Autodesk Fusion 360 part; units mm, degrees
(part 3 of 6)
ref_plane "WorkPlane5" through (73.27, 0, 0) normal (1, 0, 0) x (0, 1, 0) in component "USB — removable metal faceplate — local 1.80 mm seat"
sketch "GCT 9.64 x 3.86 gasket seat R1.65 profile" plane through (73.27, 0, 0) normal (1, 0, 0) x (0, 0, -1) in component "USB — removable metal faceplate — local 1.80 mm seat"
  line L0 (-25.07, 12.83) -> (-25.07, 19.17)
  arc A0 (-25.07, 19.17) -> (-26.72, 20.82) centre (-26.72, 19.17) ccw
  line L1 (-26.72, 20.82) -> (-27.28, 20.82)
  arc A1 (-27.28, 20.82) -> (-28.93, 19.17) centre (-27.28, 19.17) ccw
  line L2 (-28.93, 19.17) -> (-28.93, 12.83)
  arc A2 (-28.93, 12.83) -> (-27.28, 11.18) centre (-27.28, 12.83) ccw
  line L3 (-27.28, 11.18) -> (-26.72, 11.18)
  arc A3 (-26.72, 11.18) -> (-25.07, 12.83) centre (-26.72, 12.83) ccw
extrude "GCT 9.64 x 3.86 gasket seat R1.65" cut sketch "GCT 9.64 x 3.86 gasket seat R1.65 profile" along normal blind 0.5 bodies 36 in component "USB — removable metal faceplate — local 1.80 mm seat"
ref_plane "WorkPlane6" through (73.77, 0, 0) normal (1, 0, 0) x (0, 1, 0) in component "USB — removable metal faceplate — local 1.80 mm seat"
sketch "GCT throat at 0.67 mm from inner panel" plane through (73.77, 0, 0) normal (1, 0, 0) x (0, 0, -1) in component "USB — removable metal faceplate — local 1.80 mm seat"
  line L0 (-25.67, 12.83) -> (-25.67, 19.17)
  arc A0 (-25.67, 19.17) -> (-26.72, 20.22) centre (-26.72, 19.17) ccw
  line L1 (-26.72, 20.22) -> (-27.28, 20.22)
  arc A1 (-27.28, 20.22) -> (-28.33, 19.17) centre (-27.28, 19.17) ccw
  line L2 (-28.33, 19.17) -> (-28.33, 12.83)
  arc A2 (-28.33, 12.83) -> (-27.28, 11.78) centre (-27.28, 12.83) ccw
  line L3 (-27.28, 11.78) -> (-26.72, 11.78)
  arc A3 (-26.72, 11.78) -> (-25.67, 12.83) centre (-26.72, 12.83) ccw
ref_plane "WorkPlane7" through (74.9, 0, 0) normal (1, 0, 0) x (0, 1, 0) in component "USB — removable metal faceplate — local 1.80 mm seat"
sketch "GCT nominal 10-degree external lead-in" plane through (74.9, 0, 0) normal (1, 0, 0) x (0, 0, -1) in component "USB — removable metal faceplate — local 1.80 mm seat"
  line L0 (-25.4708, 12.83) -> (-25.4708, 19.17)
  arc A0 (-25.4708, 19.17) -> (-26.72, 20.4192) centre (-26.72, 19.17) ccw
  line L1 (-26.72, 20.4192) -> (-27.28, 20.4192)
  arc A1 (-27.28, 20.4192) -> (-28.5292, 19.17) centre (-27.28, 19.17) ccw
  line L2 (-28.5292, 19.17) -> (-28.5292, 12.83)
  arc A2 (-28.5292, 12.83) -> (-27.28, 11.5808) centre (-27.28, 12.83) ccw
  line L3 (-27.28, 11.5808) -> (-26.72, 11.5808)
  arc A3 (-26.72, 11.5808) -> (-25.4708, 12.83) centre (-26.72, 12.83) ccw
loft "GCT reference tapered entry cutting tool" add profiles "GCT throat at 0.67 mm from inner panel", "GCT nominal 10-degree external lead-in" section 1 section 2 separate body makes body 38 in component "USB — removable metal faceplate — local 1.80 mm seat"
combine "Nominal 10-degree USB entry" operation cut target body 36 tool bodies 38 in component "USB — removable metal faceplate — local 1.80 mm seat"
ref_plane "WorkPlane3" through (0, 0, 22.7) normal (0, 0, 1) x (1, 0, 0) in component "USB — removable panel insert and board supports"
sketch "USB board support rail sketch" plane through (0, 0, 22.7) normal (0, 0, 1) x (1, 0, 0) in component "USB — removable panel insert and board supports"
  line L0 (60.1, 8) -> (70.6, 8)
  line L1 (70.6, 8) -> (70.6, 11.6)
  line L2 (70.6, 11.6) -> (60.1, 11.6)
  line L3 (60.1, 11.6) -> (60.1, 8)
  dimension "d962" = 60.1
  dimension "d963" = 8
  dimension "d964" = 10.5
  dimension "d965" = 3.6
  constraint horizontal L0
  constraint vertical L1
  constraint horizontal L2
  constraint vertical L3
  measures "d962" horizontal distance of origin L0.start
  measures "d963" vertical distance of origin L0.start
  measures "d964" horizontal distance of L0.start L0.end
  measures "d965" vertical distance of L0.end L1.end
extrude "USB board support rail" add sketch "USB board support rail sketch" along normal blind 4 bodies 37 in component "USB — removable panel insert and board supports"
ref_plane "WorkPlane4" through (0, 0, 22.7) normal (0, 0, 1) x (1, 0, 0) in component "USB — removable panel insert and board supports"
sketch "USB board M2 support boss sketch" plane through (0, 0, 22.7) normal (0, 0, 1) x (1, 0, 0) in component "USB — removable panel insert and board supports"
  circle A0 centre (63.7, 10.4) radius 3.6
  dimension "d970" = 63.7
  dimension "d971" = 10.4
  dimension "d972" = 3.6
  measures "d970" horizontal distance of origin A0.centre
  measures "d971" vertical distance of origin A0.centre
  measures "d972" radius of A0
extrude "USB board M2 support boss" add sketch "USB board M2 support boss sketch" along normal blind 4 bodies 37 in component "USB — removable panel insert and board supports"
ref_plane "WorkPlane5" through (0, 0, 22.6) normal (0, 0, 1) x (1, 0, 0) in component "USB — removable panel insert and board supports"
sketch "USB board insert pilot reference sketch" plane through (0, 0, 22.6) normal (0, 0, 1) x (1, 0, 0) in component "USB — removable panel insert and board supports"
  circle A0 centre (63.7, 10.4) radius 1.6
  dimension "d977" = 63.7
  dimension "d978" = 10.4
  dimension "d979" = 1.6
  measures "d977" horizontal distance of origin A0.centre
  measures "d978" vertical distance of origin A0.centre
  measures "d979" radius of A0
extrude "USB board insert pilot reference" cut sketch "USB board insert pilot reference sketch" along normal blind 4.2 bodies 37 in component "USB — removable panel insert and board supports"
ref_plane "WorkPlane6" through (0, 0, 22.7) normal (0, 0, 1) x (1, 0, 0) in component "USB — removable panel insert and board supports"
sketch "USB board support rail sketch (1)" plane through (0, 0, 22.7) normal (0, 0, 1) x (1, 0, 0) in component "USB — removable panel insert and board supports"
  line L0 (57.5, 20.4) -> (70.6, 20.4)
  line L1 (70.6, 20.4) -> (70.6, 24)
  line L2 (70.6, 24) -> (57.5, 24)
  line L3 (57.5, 24) -> (57.5, 20.4)
  dimension "d984" = 57.5
  dimension "d985" = 20.4
  dimension "d986" = 13.1
  dimension "d987" = 3.6
  constraint horizontal L0
  constraint vertical L1
  constraint horizontal L2
  constraint vertical L3
  measures "d984" horizontal distance of origin L0.start
  measures "d985" vertical distance of origin L0.start
  measures "d986" horizontal distance of L0.start L0.end
  measures "d987" vertical distance of L0.end L1.end
extrude "USB board support rail (1)" add sketch "USB board support rail sketch (1)" along normal blind 4 bodies 37 in component "USB — removable panel insert and board supports"
ref_plane "WorkPlane7" through (0, 0, 22.7) normal (0, 0, 1) x (1, 0, 0) in component "USB — removable panel insert and board supports"
sketch "USB board M2 support boss sketch (1)" plane through (0, 0, 22.7) normal (0, 0, 1) x (1, 0, 0) in component "USB — removable panel insert and board supports"
  circle A0 centre (59.5, 21.6) radius 3.6
  dimension "d992" = 59.5
  dimension "d993" = 21.6
  dimension "d994" = 3.6
  measures "d992" horizontal distance of origin A0.centre
  measures "d993" vertical distance of origin A0.centre
  measures "d994" radius of A0
extrude "USB board M2 support boss (1)" add sketch "USB board M2 support boss sketch (1)" along normal blind 4 bodies 37 in component "USB — removable panel insert and board supports"
ref_plane "WorkPlane8" through (0, 0, 22.6) normal (0, 0, 1) x (1, 0, 0) in component "USB — removable panel insert and board supports"
sketch "USB board insert pilot reference sketch (1)" plane through (0, 0, 22.6) normal (0, 0, 1) x (1, 0, 0) in component "USB — removable panel insert and board supports"
  circle A0 centre (59.5, 21.6) radius 1.6
  dimension "d999" = 59.5
  dimension "d1000" = 21.6
  dimension "d1001" = 1.6
  measures "d999" horizontal distance of origin A0.centre
  measures "d1000" vertical distance of origin A0.centre
  measures "d1001" radius of A0
extrude "USB board insert pilot reference (1)" cut sketch "USB board insert pilot reference sketch (1)" along normal blind 4.2 bodies 37 in component "USB — removable panel insert and board supports"
ref_plane "WorkPlane9" through (68.6, 0, 0) normal (1, 0, 0) x (0, 1, 0) in component "USB — removable panel insert and board supports"
sketch "Metal panel M2 printed support boss sketch" plane through (68.6, 0, 0) normal (1, 0, 0) x (0, 0, -1) in component "USB — removable panel insert and board supports"
  circle A0 centre (-21.25, 8.25) radius 3.6
  dimension "d1006" = 21.25
  dimension "d1007" = 8.25
  dimension "d1008" = 3.6
  measures "d1006" horizontal distance of origin A0.centre
  measures "d1007" vertical distance of origin A0.centre
  measures "d1008" radius of A0
extrude "Metal panel M2 printed support boss" add sketch "Metal panel M2 printed support boss sketch" along normal blind 4 bodies 37 in component "USB — removable panel insert and board supports"
ref_plane "WorkPlane10" through (68.5, 0, 0) normal (1, 0, 0) x (0, 1, 0) in component "USB — removable panel insert and board supports"
sketch "Metal panel insert pilot reference sketch" plane through (68.5, 0, 0) normal (1, 0, 0) x (0, 0, -1) in component "USB — removable panel insert and board supports"
  circle A0 centre (-21.25, 8.25) radius 1.6
  dimension "d1013" = 21.25
  dimension "d1014" = 8.25
  dimension "d1015" = 1.6
  measures "d1013" horizontal distance of origin A0.centre
  measures "d1014" vertical distance of origin A0.centre
  measures "d1015" radius of A0
extrude "Metal panel insert pilot reference" cut sketch "Metal panel insert pilot reference sketch" along normal blind 4.2 bodies 37 in component "USB — removable panel insert and board supports"
ref_plane "WorkPlane8" through (72.5, 0, 0) normal (1, 0, 0) x (0, 1, 0) in component "USB — removable metal faceplate — local 1.80 mm seat"
sketch "Metal panel M2 clearance sketch" plane through (72.5, 0, 0) normal (1, 0, 0) x (0, 0, -1) in component "USB — removable metal faceplate — local 1.80 mm seat"
  circle A0 centre (-21.25, 8.25) radius 1.1
  dimension "d1020" = 21.25
  dimension "d1021" = 8.25
  dimension "d1022" = 1.1
  measures "d1020" horizontal distance of origin A0.centre
  measures "d1021" vertical distance of origin A0.centre
  measures "d1022" radius of A0
extrude "Metal panel M2 clearance" cut sketch "Metal panel M2 clearance sketch" along normal blind 2.5 bodies 36 in component "USB — removable metal faceplate — local 1.80 mm seat"
ref_plane "WorkPlane11" through (68.6, 0, 0) normal (1, 0, 0) x (0, 1, 0) in component "USB — removable panel insert and board supports"
sketch "Metal panel M2 printed support boss sketch (1)" plane through (68.6, 0, 0) normal (1, 0, 0) x (0, 0, -1) in component "USB — removable panel insert and board supports"
  circle A0 centre (-30.95, 23.75) radius 3.6
  dimension "d1027" = 30.95
  dimension "d1028" = 23.75
  dimension "d1029" = 3.6
  measures "d1027" horizontal distance of origin A0.centre
  measures "d1028" vertical distance of origin A0.centre
  measures "d1029" radius of A0
extrude "Metal panel M2 printed support boss (1)" add sketch "Metal panel M2 printed support boss sketch (1)" along normal blind 4 bodies 37 in component "USB — removable panel insert and board supports"
ref_plane "WorkPlane12" through (68.5, 0, 0) normal (1, 0, 0) x (0, 1, 0) in component "USB — removable panel insert and board supports"
sketch "Metal panel insert pilot reference sketch (1)" plane through (68.5, 0, 0) normal (1, 0, 0) x (0, 0, -1) in component "USB — removable panel insert and board supports"
  circle A0 centre (-30.95, 23.75) radius 1.6
  dimension "d1034" = 30.95
  dimension "d1035" = 23.75
  dimension "d1036" = 1.6
  measures "d1034" horizontal distance of origin A0.centre
  measures "d1035" vertical distance of origin A0.centre
  measures "d1036" radius of A0
extrude "Metal panel insert pilot reference (1)" cut sketch "Metal panel insert pilot reference sketch (1)" along normal blind 4.2 bodies 37 in component "USB — removable panel insert and board supports"
ref_plane "WorkPlane9" through (72.5, 0, 0) normal (1, 0, 0) x (0, 1, 0) in component "USB — removable metal faceplate — local 1.80 mm seat"
sketch "Metal panel M2 clearance sketch (1)" plane through (72.5, 0, 0) normal (1, 0, 0) x (0, 0, -1) in component "USB — removable metal faceplate — local 1.80 mm seat"
  circle A0 centre (-30.95, 23.75) radius 1.1
  dimension "d1041" = 30.95
  dimension "d1042" = 23.75
  dimension "d1043" = 1.1
  measures "d1041" horizontal distance of origin A0.centre
  measures "d1042" vertical distance of origin A0.centre
  measures "d1043" radius of A0
extrude "Metal panel M2 clearance (1)" cut sketch "Metal panel M2 clearance sketch (1)" along normal blind 2.5 bodies 36 in component "USB — removable metal faceplate — local 1.80 mm seat"
ref_plane "WorkPlane1" through (0, 0, 26.7) normal (0, 0, 1) x (1, 0, 0) in component "USB — 0.60 mm daughterboard — layout provisional"
sketch "USB 0.60 mm daughterboard sketch" plane through (0, 0, 26.7) normal (0, 0, 1) x (1, 0, 0) in component "USB — 0.60 mm daughterboard — layout provisional"
  line L0 (57, 8) -> (70.6, 8)
  line L1 (70.6, 8) -> (70.6, 24)
  line L2 (70.6, 24) -> (57, 24)
  line L3 (57, 24) -> (57, 8)
  dimension "d1048" = 57
  dimension "d1049" = 8
  dimension "d1050" = 13.6
  dimension "d1051" = 16
  constraint horizontal L0
  constraint vertical L1
  constraint horizontal L2
  constraint vertical L3
  measures "d1048" horizontal distance of origin L0.start
  measures "d1049" vertical distance of origin L0.start
  measures "d1050" horizontal distance of L0.start L0.end
  measures "d1051" vertical distance of L0.end L1.end
extrude "USB 0.60 mm daughterboard" add sketch "USB 0.60 mm daughterboard sketch" along normal blind 0.6 separate body makes body 39 in component "USB — 0.60 mm daughterboard — layout provisional"
ref_plane "WorkPlane2" through (0, 0, 26.6) normal (0, 0, 1) x (1, 0, 0) in component "USB — 0.60 mm daughterboard — layout provisional"
sketch "Sketch2" plane through (0, 0, 26.6) normal (0, 0, 1) x (1, 0, 0) in component "USB — 0.60 mm daughterboard — layout provisional"
  line L0 (66.3, 11.37) -> (70.7, 11.37)
  line L1 (70.7, 11.37) -> (70.7, 20.63)
  line L2 (70.7, 20.63) -> (66.3, 20.63)
  line L3 (66.3, 20.63) -> (66.3, 11.37)
  dimension "d1056" = 66.3
  dimension "d1057" = 11.37
  dimension "d1058" = 4.4
  dimension "d1059" = 9.26
  constraint horizontal L0
  constraint vertical L1
  constraint horizontal L2
  constraint vertical L3
  measures "d1056" horizontal distance of origin L0.start
  measures "d1057" vertical distance of origin L0.start
  measures "d1058" horizontal distance of L0.start L0.end
  measures "d1059" vertical distance of L0.end L1.end
extrude "Connector straddle clearance — footprint to reconcile" cut sketch "Sketch2" along normal blind 0.8 bodies 39 in component "USB — 0.60 mm daughterboard — layout provisional"
ref_plane "WorkPlane3" through (0, 0, 26.6) normal (0, 0, 1) x (1, 0, 0) in component "USB — 0.60 mm daughterboard — layout provisional"
sketch "M2 daughterboard clearance sketch" plane through (0, 0, 26.6) normal (0, 0, 1) x (1, 0, 0) in component "USB — 0.60 mm daughterboard — layout provisional"
  circle A0 centre (63.7, 10.4) radius 1.1
  dimension "d1064" = 63.7
  dimension "d1065" = 10.4
  dimension "d1066" = 1.1
  measures "d1064" horizontal distance of origin A0.centre
  measures "d1065" vertical distance of origin A0.centre
  measures "d1066" radius of A0
extrude "M2 daughterboard clearance" cut sketch "M2 daughterboard clearance sketch" along normal blind 0.8 bodies 39 in component "USB — 0.60 mm daughterboard — layout provisional"
ref_plane "WorkPlane4" through (0, 0, 26.6) normal (0, 0, 1) x (1, 0, 0) in component "USB — 0.60 mm daughterboard — layout provisional"
sketch "M2 daughterboard clearance sketch (1)" plane through (0, 0, 26.6) normal (0, 0, 1) x (1, 0, 0) in component "USB — 0.60 mm daughterboard — layout provisional"
  circle A0 centre (59.5, 21.6) radius 1.1
  dimension "d1071" = 59.5
  dimension "d1072" = 21.6
  dimension "d1073" = 1.1
  measures "d1071" horizontal distance of origin A0.centre
  measures "d1072" vertical distance of origin A0.centre
  measures "d1073" radius of A0
extrude "M2 daughterboard clearance (1)" cut sketch "M2 daughterboard clearance sketch (1)" along normal blind 0.8 bodies 39 in component "USB — 0.60 mm daughterboard — layout provisional"
ref_plane "WorkPlane1" through (67.5, 0, 0) normal (1, 0, 0) x (0, 1, 0) in component "USB — GCT USB4720 metal shell — drawing reconstruction"
sketch "USB stainless shell body reference profile" plane through (67.5, 0, 0) normal (1, 0, 0) x (0, 0, -1) in component "USB — GCT USB4720 metal shell — drawing reconstruction"
  line L0 (-25.37, 12.88) -> (-25.37, 19.12)
  arc A0 (-25.37, 19.12) -> (-26.42, 20.17) centre (-26.42, 19.12) ccw
  line L1 (-26.42, 20.17) -> (-27.58, 20.17)
  arc A1 (-27.58, 20.17) -> (-28.63, 19.12) centre (-27.58, 19.12) ccw
  line L2 (-28.63, 19.12) -> (-28.63, 12.88)
  arc A2 (-28.63, 12.88) -> (-27.58, 11.83) centre (-27.58, 12.88) ccw
  line L3 (-27.58, 11.83) -> (-26.42, 11.83)
  arc A3 (-26.42, 11.83) -> (-25.37, 12.88) centre (-26.42, 12.88) ccw
extrude "USB stainless shell body reference" add sketch "USB stainless shell body reference profile" along normal blind 5.4 separate body makes body 40 in component "USB — GCT USB4720 metal shell — drawing reconstruction"
ref_plane "WorkPlane2" through (72.9, 0, 0) normal (1, 0, 0) x (0, 1, 0) in component "USB — GCT USB4720 metal shell — drawing reconstruction"
sketch "USB nose 8.34 x 2.56 reference profile" plane through (72.9, 0, 0) normal (1, 0, 0) x (0, 0, -1) in component "USB — GCT USB4720 metal shell — drawing reconstruction"
  line L0 (-25.72, 12.88) -> (-25.72, 19.12)
  arc A0 (-25.72, 19.12) -> (-26.77, 20.17) centre (-26.77, 19.12) ccw
  line L1 (-26.77, 20.17) -> (-27.23, 20.17)
  arc A1 (-27.23, 20.17) -> (-28.28, 19.12) centre (-27.23, 19.12) ccw
  line L2 (-28.28, 19.12) -> (-28.28, 12.88)
  arc A2 (-28.28, 12.88) -> (-27.23, 11.83) centre (-27.23, 12.88) ccw
  line L3 (-27.23, 11.83) -> (-26.77, 11.83)
  arc A3 (-26.77, 11.83) -> (-25.72, 12.88) centre (-26.77, 12.88) ccw
extrude "USB nose 8.34 x 2.56 reference" add sketch "USB nose 8.34 x 2.56 reference profile" along normal blind 1.1 bodies 40 in component "USB — GCT USB4720 metal shell — drawing reconstruction"
ref_plane "WorkPlane3" through (67.4, 0, 0) normal (1, 0, 0) x (0, 1, 0) in component "USB — GCT USB4720 metal shell — drawing reconstruction"
sketch "Sketch3" plane through (67.4, 0, 0) normal (1, 0, 0) x (0, 0, -1) in component "USB — GCT USB4720 metal shell — drawing reconstruction"
  line L0 (-25.57, 12.88) -> (-25.57, 19.12)
  arc A0 (-25.57, 19.12) -> (-26.42, 19.97) centre (-26.42, 19.12) ccw
  line L1 (-26.42, 19.97) -> (-27.58, 19.97)
  arc A1 (-27.58, 19.97) -> (-28.43, 19.12) centre (-27.58, 19.12) ccw
  line L2 (-28.43, 19.12) -> (-28.43, 12.88)
  arc A2 (-28.43, 12.88) -> (-27.58, 12.03) centre (-27.58, 12.88) ccw
  line L3 (-27.58, 12.03) -> (-26.42, 12.03)
  arc A3 (-26.42, 12.03) -> (-25.57, 12.88) centre (-26.42, 12.88) ccw
extrude "Shell rear cavity — illustrative wall" cut sketch "Sketch3" along normal blind 5.5 bodies 40 in component "USB — GCT USB4720 metal shell — drawing reconstruction"
ref_plane "WorkPlane4" through (72.8, 0, 0) normal (1, 0, 0) x (0, 1, 0) in component "USB — GCT USB4720 metal shell — drawing reconstruction"
sketch "Sketch4" plane through (72.8, 0, 0) normal (1, 0, 0) x (0, 0, -1) in component "USB — GCT USB4720 metal shell — drawing reconstruction"
  line L0 (-25.92, 12.88) -> (-25.92, 19.12)
  arc A0 (-25.92, 19.12) -> (-26.77, 19.97) centre (-26.77, 19.12) ccw
  line L1 (-26.77, 19.97) -> (-27.23, 19.97)
  arc A1 (-27.23, 19.97) -> (-28.08, 19.12) centre (-27.23, 19.12) ccw
  line L2 (-28.08, 19.12) -> (-28.08, 12.88)
  arc A2 (-28.08, 12.88) -> (-27.23, 12.03) centre (-27.23, 12.88) ccw
  line L3 (-27.23, 12.03) -> (-26.77, 12.03)
  arc A3 (-26.77, 12.03) -> (-25.92, 12.88) centre (-26.77, 12.88) ccw
extrude "Mating shell opening — illustrative wall" cut sketch "Sketch4" along normal blind 1.3 bodies 40 in component "USB — GCT USB4720 metal shell — drawing reconstruction"
ref_plane "WorkPlane5" through (0, 0, 27.3) normal (0, 0, 1) x (1, 0, 0) in component "USB — GCT USB4720 metal shell — drawing reconstruction"
sketch "Sketch5" plane through (0, 0, 27.3) normal (0, 0, 1) x (1, 0, 0) in component "USB — GCT USB4720 metal shell — drawing reconstruction"
  line L0 (67.8, 10.35) -> (69.1, 10.35)
  line L1 (69.1, 10.35) -> (69.1, 11.88)
  line L2 (69.1, 11.88) -> (67.8, 11.88)
  line L3 (67.8, 11.88) -> (67.8, 10.35)
  dimension "d1094" = 67.8
  dimension "d1095" = 10.35
  dimension "d1096" = 1.3
  dimension "d1097" = 1.53
  constraint horizontal L0
  constraint vertical L1
  constraint horizontal L2
  constraint vertical L3
  measures "d1094" horizontal distance of origin L0.start
  measures "d1095" vertical distance of origin L0.start
  measures "d1096" horizontal distance of L0.start L0.end
  measures "d1097" vertical distance of L0.end L1.end
extrude "Grounding wing — placement illustrative" add sketch "Sketch5" along normal blind 0.3 bodies 40 in component "USB — GCT USB4720 metal shell — drawing reconstruction"
ref_plane "WorkPlane6" through (0, 0, 27.3) normal (0, 0, 1) x (1, 0, 0) in component "USB — GCT USB4720 metal shell — drawing reconstruction"
sketch "Sketch6" plane through (0, 0, 27.3) normal (0, 0, 1) x (1, 0, 0) in component "USB — GCT USB4720 metal shell — drawing reconstruction"
  line L0 (67.8, 20.12) -> (69.1, 20.12)
  line L1 (69.1, 20.12) -> (69.1, 21.65)
  line L2 (69.1, 21.65) -> (67.8, 21.65)
  line L3 (67.8, 21.65) -> (67.8, 20.12)
  dimension "d1102" = 67.8
  dimension "d1103" = 20.12
  dimension "d1104" = 1.3
  dimension "d1105" = 1.53
  constraint horizontal L0
  constraint vertical L1
  constraint horizontal L2
  constraint vertical L3
  measures "d1102" horizontal distance of origin L0.start
  measures "d1103" vertical distance of origin L0.start
  measures "d1104" horizontal distance of L0.start L0.end
  measures "d1105" vertical distance of L0.end L1.end
extrude "Grounding wing — placement illustrative (1)" add sketch "Sketch6" along normal blind 0.3 bodies 40 in component "USB — GCT USB4720 metal shell — drawing reconstruction"
ref_plane "WorkPlane7" through (0, 0, 27.3) normal (0, 0, 1) x (1, 0, 0) in component "USB — GCT USB4720 metal shell — drawing reconstruction"
sketch "Sketch7" plane through (0, 0, 27.3) normal (0, 0, 1) x (1, 0, 0) in component "USB — GCT USB4720 metal shell — drawing reconstruction"
  line L0 (69.8, 10.35) -> (71.1, 10.35)
  line L1 (71.1, 10.35) -> (71.1, 11.88)
  line L2 (71.1, 11.88) -> (69.8, 11.88)
  line L3 (69.8, 11.88) -> (69.8, 10.35)
  dimension "d1110" = 69.8
  dimension "d1111" = 10.35
  dimension "d1112" = 1.3
  dimension "d1113" = 1.53
  constraint horizontal L0
  constraint vertical L1
  constraint horizontal L2
  constraint vertical L3
  measures "d1110" horizontal distance of origin L0.start
  measures "d1111" vertical distance of origin L0.start
  measures "d1112" horizontal distance of L0.start L0.end
  measures "d1113" vertical distance of L0.end L1.end
extrude "Grounding wing — placement illustrative (2)" add sketch "Sketch7" along normal blind 0.3 bodies 40 in component "USB — GCT USB4720 metal shell — drawing reconstruction"
ref_plane "WorkPlane8" through (0, 0, 27.3) normal (0, 0, 1) x (1, 0, 0) in component "USB — GCT USB4720 metal shell — drawing reconstruction"
sketch "Sketch8" plane through (0, 0, 27.3) normal (0, 0, 1) x (1, 0, 0) in component "USB — GCT USB4720 metal shell — drawing reconstruction"
  line L0 (69.8, 20.12) -> (71.1, 20.12)
  line L1 (71.1, 20.12) -> (71.1, 21.65)
  line L2 (71.1, 21.65) -> (69.8, 21.65)
  line L3 (69.8, 21.65) -> (69.8, 20.12)
  dimension "d1118" = 69.8
  dimension "d1119" = 20.12
  dimension "d1120" = 1.3
  dimension "d1121" = 1.53
  constraint horizontal L0
  constraint vertical L1
  constraint horizontal L2
  constraint vertical L3
  measures "d1118" horizontal distance of origin L0.start
  measures "d1119" vertical distance of origin L0.start
  measures "d1120" horizontal distance of L0.start L0.end
  measures "d1121" vertical distance of L0.end L1.end
extrude "Grounding wing — placement illustrative (3)" add sketch "Sketch8" along normal blind 0.3 bodies 40 in component "USB — GCT USB4720 metal shell — drawing reconstruction"
ref_plane "WorkPlane1" through (67.4, 0, 0) normal (1, 0, 0) x (0, 1, 0) in component "USB — GCT tongue and rear insulator — illustrative"
sketch "Sketch1" plane through (67.4, 0, 0) normal (1, 0, 0) x (0, 0, -1) in component "USB — GCT tongue and rear insulator — illustrative"
  line L0 (-25.95, 12.6) -> (-25.95, 19.4)
  arc A0 (-25.95, 19.4) -> (-26.45, 19.9) centre (-26.45, 19.4) ccw
  line L1 (-26.45, 19.9) -> (-27.55, 19.9)
  arc A1 (-27.55, 19.9) -> (-28.05, 19.4) centre (-27.55, 19.4) ccw
  line L2 (-28.05, 19.4) -> (-28.05, 12.6)
  arc A2 (-28.05, 12.6) -> (-27.55, 12.1) centre (-27.55, 12.6) ccw
  line L3 (-27.55, 12.1) -> (-26.45, 12.1)
  arc A3 (-26.45, 12.1) -> (-25.95, 12.6) centre (-26.45, 12.6) ccw
extrude "Insulator rear block — visual reference" add sketch "Sketch1" along normal blind 1 separate body makes body 41 in component "USB — GCT tongue and rear insulator — illustrative"
ref_plane "WorkPlane2" through (0, 0, 26.65) normal (0, 0, 1) x (1, 0, 0) in component "USB — GCT tongue and rear insulator — illustrative"
sketch "Sketch2 (2)" plane through (0, 0, 26.65) normal (0, 0, 1) x (1, 0, 0) in component "USB — GCT tongue and rear insulator — illustrative"
  line L0 (68.4, 12.655) -> (73.8, 12.655)
  line L1 (73.8, 12.655) -> (73.8, 19.345)
  line L2 (73.8, 19.345) -> (68.4, 19.345)
  line L3 (68.4, 19.345) -> (68.4, 12.655)
  dimension "d1130" = 68.4
  dimension "d1131" = 12.655
  dimension "d1132" = 5.4
  dimension "d1133" = 6.69
  constraint horizontal L0
  constraint vertical L1
  constraint horizontal L2
  constraint vertical L3
  measures "d1130" horizontal distance of origin L0.start
  measures "d1131" vertical distance of origin L0.start
  measures "d1132" horizontal distance of L0.start L0.end
  measures "d1133" vertical distance of L0.end L1.end
extrude "USB tongue — 6.69 x 0.70 nominal reference" add sketch "Sketch2 (2)" along normal blind 0.7 bodies 41 in component "USB — GCT tongue and rear insulator — illustrative"
ref_plane "WorkPlane1" through (73.3, 0, 0) normal (1, 0, 0) x (0, 1, 0) in component "USB — GCT LIM gasket — drawing reference"
sketch "LIM gasket nominal reference profile" plane through (73.3, 0, 0) normal (1, 0, 0) x (0, 0, -1) in component "USB — GCT LIM gasket — drawing reference"
  line L0 (-25.14, 12.75) -> (-25.14, 19.25)
  arc A0 (-25.14, 19.25) -> (-26.64, 20.75) centre (-26.64, 19.25) ccw
  line L1 (-26.64, 20.75) -> (-27.36, 20.75)
  arc A1 (-27.36, 20.75) -> (-28.86, 19.25) centre (-27.36, 19.25) ccw
  line L2 (-28.86, 19.25) -> (-28.86, 12.75)
  arc A2 (-28.86, 12.75) -> (-27.36, 11.25) centre (-27.36, 12.75) ccw
  line L3 (-27.36, 11.25) -> (-26.64, 11.25)
  arc A3 (-26.64, 11.25) -> (-25.14, 12.75) centre (-26.64, 12.75) ccw
extrude "LIM gasket nominal reference" add sketch "LIM gasket nominal reference profile" along normal blind 0.4 separate body makes body 42 in component "USB — GCT LIM gasket — drawing reference"
ref_plane "WorkPlane2" through (73.29, 0, 0) normal (1, 0, 0) x (0, 1, 0) in component "USB — GCT LIM gasket — drawing reference"
sketch "Gasket shell clearance profile" plane through (73.29, 0, 0) normal (1, 0, 0) x (0, 0, -1) in component "USB — GCT LIM gasket — drawing reference"
  line L0 (-25.7, 12.88) -> (-25.7, 19.12)
  arc A0 (-25.7, 19.12) -> (-26.77, 20.19) centre (-26.77, 19.12) ccw
  line L1 (-26.77, 20.19) -> (-27.23, 20.19)
  arc A1 (-27.23, 20.19) -> (-28.3, 19.12) centre (-27.23, 19.12) ccw
  line L2 (-28.3, 19.12) -> (-28.3, 12.88)
  arc A2 (-28.3, 12.88) -> (-27.23, 11.81) centre (-27.23, 12.88) ccw
  line L3 (-27.23, 11.81) -> (-26.77, 11.81)
  arc A3 (-26.77, 11.81) -> (-25.7, 12.88) centre (-26.77, 12.88) ccw
extrude "Gasket shell clearance" cut sketch "Gasket shell clearance profile" along normal blind 0.42 bodies 42 in component "USB — GCT LIM gasket — drawing reference"
ref_plane "WorkPlane1" through (0, 0, 26.62) normal (0, 0, 1) x (1, 0, 0) in component "USB — contact detail — illustrative only"
sketch "USB contact visual stripe sketch" plane through (0, 0, 26.62) normal (0, 0, 1) x (1, 0, 0) in component "USB — contact detail — illustrative only"
  line L0 (71, 14.125) -> (73.7, 14.125)
  line L1 (73.7, 14.125) -> (73.7, 14.375)
  line L2 (73.7, 14.375) -> (71, 14.375)
  line L3 (71, 14.375) -> (71, 14.125)
  dimension "d1146" = 71
  dimension "d1147" = 14.125
  dimension "d1148" = 2.7
  dimension "d1149" = 0.25
  constraint horizontal L0
  constraint vertical L1
  constraint horizontal L2
  constraint vertical L3
  measures "d1146" horizontal distance of origin L0.start
  measures "d1147" vertical distance of origin L0.start
  measures "d1148" horizontal distance of L0.start L0.end
  measures "d1149" vertical distance of L0.end L1.end
extrude "USB contact visual stripe" add sketch "USB contact visual stripe sketch" along normal blind 0.03 separate body makes body 43 in component "USB — contact detail — illustrative only"
ref_plane "WorkPlane2" through (0, 0, 26.62) normal (0, 0, 1) x (1, 0, 0) in component "USB — contact detail — illustrative only"
sketch "USB contact visual stripe sketch (1)" plane through (0, 0, 26.62) normal (0, 0, 1) x (1, 0, 0) in component "USB — contact detail — illustrative only"
  line L0 (71, 14.625) -> (73.7, 14.625)
  line L1 (73.7, 14.625) -> (73.7, 14.875)
  line L2 (73.7, 14.875) -> (71, 14.875)
  line L3 (71, 14.875) -> (71, 14.625)
  dimension "d1154" = 71
  dimension "d1155" = 14.625
  dimension "d1156" = 2.7
  dimension "d1157" = 0.25
  constraint horizontal L0
  constraint vertical L1
  constraint horizontal L2
  constraint vertical L3
  measures "d1154" horizontal distance of origin L0.start
  measures "d1155" vertical distance of origin L0.start
  measures "d1156" horizontal distance of L0.start L0.end
  measures "d1157" vertical distance of L0.end L1.end
extrude "USB contact visual stripe (1)" add sketch "USB contact visual stripe sketch (1)" along normal blind 0.03 separate body makes body 44 in component "USB — contact detail — illustrative only"
ref_plane "WorkPlane3" through (0, 0, 26.62) normal (0, 0, 1) x (1, 0, 0) in component "USB — contact detail — illustrative only"
sketch "USB contact visual stripe sketch (2)" plane through (0, 0, 26.62) normal (0, 0, 1) x (1, 0, 0) in component "USB — contact detail — illustrative only"
  line L0 (71, 15.125) -> (73.7, 15.125)
  line L1 (73.7, 15.125) -> (73.7, 15.375)
  line L2 (73.7, 15.375) -> (71, 15.375)
  line L3 (71, 15.375) -> (71, 15.125)
  dimension "d1162" = 71
  dimension "d1163" = 15.125
  dimension "d1164" = 2.7
  dimension "d1165" = 0.25
  constraint horizontal L0
  constraint vertical L1
  constraint horizontal L2
  constraint vertical L3
  measures "d1162" horizontal distance of origin L0.start
  measures "d1163" vertical distance of origin L0.start
  measures "d1164" horizontal distance of L0.start L0.end
  measures "d1165" vertical distance of L0.end L1.end
extrude "USB contact visual stripe (2)" add sketch "USB contact visual stripe sketch (2)" along normal blind 0.03 separate body makes body 45 in component "USB — contact detail — illustrative only"
ref_plane "WorkPlane4" through (0, 0, 26.62) normal (0, 0, 1) x (1, 0, 0) in component "USB — contact detail — illustrative only"
sketch "USB contact visual stripe sketch (3)" plane through (0, 0, 26.62) normal (0, 0, 1) x (1, 0, 0) in component "USB — contact detail — illustrative only"
  line L0 (71, 15.625) -> (73.7, 15.625)
  line L1 (73.7, 15.625) -> (73.7, 15.875)
  line L2 (73.7, 15.875) -> (71, 15.875)
  line L3 (71, 15.875) -> (71, 15.625)
  dimension "d1170" = 71
  dimension "d1171" = 15.625
  dimension "d1172" = 2.7
  dimension "d1173" = 0.25
  constraint horizontal L0
  constraint vertical L1
  constraint horizontal L2
  constraint vertical L3
  measures "d1170" horizontal distance of origin L0.start
  measures "d1171" vertical distance of origin L0.start
  measures "d1172" horizontal distance of L0.start L0.end
  measures "d1173" vertical distance of L0.end L1.end
extrude "USB contact visual stripe (3)" add sketch "USB contact visual stripe sketch (3)" along normal blind 0.03 separate body makes body 46 in component "USB — contact detail — illustrative only"
ref_plane "WorkPlane5" through (0, 0, 26.62) normal (0, 0, 1) x (1, 0, 0) in component "USB — contact detail — illustrative only"
sketch "USB contact visual stripe sketch (4)" plane through (0, 0, 26.62) normal (0, 0, 1) x (1, 0, 0) in component "USB — contact detail — illustrative only"
  line L0 (71, 16.125) -> (73.7, 16.125)
  line L1 (73.7, 16.125) -> (73.7, 16.375)
  line L2 (73.7, 16.375) -> (71, 16.375)
  line L3 (71, 16.375) -> (71, 16.125)
  dimension "d1178" = 71
  dimension "d1179" = 16.125
  dimension "d1180" = 2.7
  dimension "d1181" = 0.25
  constraint horizontal L0
  constraint vertical L1
  constraint horizontal L2
  constraint vertical L3
  measures "d1178" horizontal distance of origin L0.start
  measures "d1179" vertical distance of origin L0.start
  measures "d1180" horizontal distance of L0.start L0.end
  measures "d1181" vertical distance of L0.end L1.end
extrude "USB contact visual stripe (4)" add sketch "USB contact visual stripe sketch (4)" along normal blind 0.03 separate body makes body 47 in component "USB — contact detail — illustrative only"
ref_plane "WorkPlane6" through (0, 0, 26.62) normal (0, 0, 1) x (1, 0, 0) in component "USB — contact detail — illustrative only"
sketch "USB contact visual stripe sketch (5)" plane through (0, 0, 26.62) normal (0, 0, 1) x (1, 0, 0) in component "USB — contact detail — illustrative only"
  line L0 (71, 16.625) -> (73.7, 16.625)
  line L1 (73.7, 16.625) -> (73.7, 16.875)
  line L2 (73.7, 16.875) -> (71, 16.875)
  line L3 (71, 16.875) -> (71, 16.625)
  dimension "d1186" = 71
  dimension "d1187" = 16.625
  dimension "d1188" = 2.7
  dimension "d1189" = 0.25
  constraint horizontal L0
  constraint vertical L1
  constraint horizontal L2
  constraint vertical L3
  measures "d1186" horizontal distance of origin L0.start
  measures "d1187" vertical distance of origin L0.start
  measures "d1188" horizontal distance of L0.start L0.end
  measures "d1189" vertical distance of L0.end L1.end
extrude "USB contact visual stripe (5)" add sketch "USB contact visual stripe sketch (5)" along normal blind 0.03 separate body makes body 48 in component "USB — contact detail — illustrative only"
ref_plane "WorkPlane7" through (0, 0, 26.62) normal (0, 0, 1) x (1, 0, 0) in component "USB — contact detail — illustrative only"
sketch "USB contact visual stripe sketch (6)" plane through (0, 0, 26.62) normal (0, 0, 1) x (1, 0, 0) in component "USB — contact detail — illustrative only"
  line L0 (71, 17.125) -> (73.7, 17.125)
  line L1 (73.7, 17.125) -> (73.7, 17.375)
  line L2 (73.7, 17.375) -> (71, 17.375)
  line L3 (71, 17.375) -> (71, 17.125)
  dimension "d1194" = 71
  dimension "d1195" = 17.125
  dimension "d1196" = 2.7
  dimension "d1197" = 0.25
  constraint horizontal L0
  constraint vertical L1
  constraint horizontal L2
  constraint vertical L3
  measures "d1194" horizontal distance of origin L0.start
  measures "d1195" vertical distance of origin L0.start
  measures "d1196" horizontal distance of L0.start L0.end
  measures "d1197" vertical distance of L0.end L1.end
extrude "USB contact visual stripe (6)" add sketch "USB contact visual stripe sketch (6)" along normal blind 0.03 separate body makes body 49 in component "USB — contact detail — illustrative only"
ref_plane "WorkPlane8" through (0, 0, 26.62) normal (0, 0, 1) x (1, 0, 0) in component "USB — contact detail — illustrative only"
sketch "USB contact visual stripe sketch (7)" plane through (0, 0, 26.62) normal (0, 0, 1) x (1, 0, 0) in component "USB — contact detail — illustrative only"
  line L0 (71, 17.625) -> (73.7, 17.625)
  line L1 (73.7, 17.625) -> (73.7, 17.875)
  line L2 (73.7, 17.875) -> (71, 17.875)
  line L3 (71, 17.875) -> (71, 17.625)
  dimension "d1202" = 71
  dimension "d1203" = 17.625
  dimension "d1204" = 2.7
  dimension "d1205" = 0.25
  constraint horizontal L0
  constraint vertical L1
  constraint horizontal L2
  constraint vertical L3
  measures "d1202" horizontal distance of origin L0.start
  measures "d1203" vertical distance of origin L0.start
  measures "d1204" horizontal distance of L0.start L0.end
  measures "d1205" vertical distance of L0.end L1.end
extrude "USB contact visual stripe (7)" add sketch "USB contact visual stripe sketch (7)" along normal blind 0.03 separate body makes body 50 in component "USB — contact detail — illustrative only"
ref_plane "WorkPlane9" through (0, 0, 27.35) normal (0, 0, 1) x (1, 0, 0) in component "USB — contact detail — illustrative only"
sketch "USB contact visual stripe sketch (8)" plane through (0, 0, 27.35) normal (0, 0, 1) x (1, 0, 0) in component "USB — contact detail — illustrative only"
  line L0 (71, 14.125) -> (73.7, 14.125)
  line L1 (73.7, 14.125) -> (73.7, 14.375)
  line L2 (73.7, 14.375) -> (71, 14.375)
  line L3 (71, 14.375) -> (71, 14.125)
  dimension "d1210" = 71
  dimension "d1211" = 14.125
  dimension "d1212" = 2.7
  dimension "d1213" = 0.25
  constraint horizontal L0
  constraint vertical L1
  constraint horizontal L2
  constraint vertical L3
  measures "d1210" horizontal distance of origin L0.start
  measures "d1211" vertical distance of origin L0.start
  measures "d1212" horizontal distance of L0.start L0.end
  measures "d1213" vertical distance of L0.end L1.end
extrude "USB contact visual stripe (8)" add sketch "USB contact visual stripe sketch (8)" along normal blind 0.03 separate body makes body 51 in component "USB — contact detail — illustrative only"
ref_plane "WorkPlane10" through (0, 0, 27.35) normal (0, 0, 1) x (1, 0, 0) in component "USB — contact detail — illustrative only"
sketch "USB contact visual stripe sketch (9)" plane through (0, 0, 27.35) normal (0, 0, 1) x (1, 0, 0) in component "USB — contact detail — illustrative only"
  line L0 (71, 14.625) -> (73.7, 14.625)
  line L1 (73.7, 14.625) -> (73.7, 14.875)
  line L2 (73.7, 14.875) -> (71, 14.875)
  line L3 (71, 14.875) -> (71, 14.625)
  dimension "d1218" = 71
  dimension "d1219" = 14.625
  dimension "d1220" = 2.7
  dimension "d1221" = 0.25
  constraint horizontal L0
  constraint vertical L1
  constraint horizontal L2
  constraint vertical L3
  measures "d1218" horizontal distance of origin L0.start
  measures "d1219" vertical distance of origin L0.start
  measures "d1220" horizontal distance of L0.start L0.end
  measures "d1221" vertical distance of L0.end L1.end
extrude "USB contact visual stripe (9)" add sketch "USB contact visual stripe sketch (9)" along normal blind 0.03 separate body makes body 52 in component "USB — contact detail — illustrative only"
ref_plane "WorkPlane11" through (0, 0, 27.35) normal (0, 0, 1) x (1, 0, 0) in component "USB — contact detail — illustrative only"
sketch "USB contact visual stripe sketch (10)" plane through (0, 0, 27.35) normal (0, 0, 1) x (1, 0, 0) in component "USB — contact detail — illustrative only"
  line L0 (71, 15.125) -> (73.7, 15.125)
  line L1 (73.7, 15.125) -> (73.7, 15.375)
  line L2 (73.7, 15.375) -> (71, 15.375)
  line L3 (71, 15.375) -> (71, 15.125)
  dimension "d1226" = 71
  dimension "d1227" = 15.125
  dimension "d1228" = 2.7
  dimension "d1229" = 0.25
  constraint horizontal L0
  constraint vertical L1
  constraint horizontal L2
  constraint vertical L3
  measures "d1226" horizontal distance of origin L0.start
  measures "d1227" vertical distance of origin L0.start
  measures "d1228" horizontal distance of L0.start L0.end
  measures "d1229" vertical distance of L0.end L1.end
extrude "USB contact visual stripe (10)" add sketch "USB contact visual stripe sketch (10)" along normal blind 0.03 separate body makes body 53 in component "USB — contact detail — illustrative only"
ref_plane "WorkPlane12" through (0, 0, 27.35) normal (0, 0, 1) x (1, 0, 0) in component "USB — contact detail — illustrative only"
sketch "USB contact visual stripe sketch (11)" plane through (0, 0, 27.35) normal (0, 0, 1) x (1, 0, 0) in component "USB — contact detail — illustrative only"
  line L0 (71, 15.625) -> (73.7, 15.625)
  line L1 (73.7, 15.625) -> (73.7, 15.875)
  line L2 (73.7, 15.875) -> (71, 15.875)
  line L3 (71, 15.875) -> (71, 15.625)
  dimension "d1234" = 71
  dimension "d1235" = 15.625
  dimension "d1236" = 2.7
  dimension "d1237" = 0.25
  constraint horizontal L0
  constraint vertical L1
  constraint horizontal L2
  constraint vertical L3
  measures "d1234" horizontal distance of origin L0.start
  measures "d1235" vertical distance of origin L0.start
  measures "d1236" horizontal distance of L0.start L0.end
  measures "d1237" vertical distance of L0.end L1.end
extrude "USB contact visual stripe (11)" add sketch "USB contact visual stripe sketch (11)" along normal blind 0.03 separate body makes body 54 in component "USB — contact detail — illustrative only"
ref_plane "WorkPlane13" through (0, 0, 27.35) normal (0, 0, 1) x (1, 0, 0) in component "USB — contact detail — illustrative only"
sketch "USB contact visual stripe sketch (12)" plane through (0, 0, 27.35) normal (0, 0, 1) x (1, 0, 0) in component "USB — contact detail — illustrative only"
  line L0 (71, 16.125) -> (73.7, 16.125)
  line L1 (73.7, 16.125) -> (73.7, 16.375)
  line L2 (73.7, 16.375) -> (71, 16.375)
  line L3 (71, 16.375) -> (71, 16.125)
  dimension "d1242" = 71
  dimension "d1243" = 16.125
  dimension "d1244" = 2.7
  dimension "d1245" = 0.25
  constraint horizontal L0
  constraint vertical L1
  constraint horizontal L2
  constraint vertical L3
  measures "d1242" horizontal distance of origin L0.start
  measures "d1243" vertical distance of origin L0.start
  measures "d1244" horizontal distance of L0.start L0.end
  measures "d1245" vertical distance of L0.end L1.end
extrude "USB contact visual stripe (12)" add sketch "USB contact visual stripe sketch (12)" along normal blind 0.03 separate body makes body 55 in component "USB — contact detail — illustrative only"
ref_plane "WorkPlane14" through (0, 0, 27.35) normal (0, 0, 1) x (1, 0, 0) in component "USB — contact detail — illustrative only"
sketch "USB contact visual stripe sketch (13)" plane through (0, 0, 27.35) normal (0, 0, 1) x (1, 0, 0) in component "USB — contact detail — illustrative only"
  line L0 (71, 16.625) -> (73.7, 16.625)
  line L1 (73.7, 16.625) -> (73.7, 16.875)
  line L2 (73.7, 16.875) -> (71, 16.875)
  line L3 (71, 16.875) -> (71, 16.625)
  dimension "d1250" = 71
  dimension "d1251" = 16.625
  dimension "d1252" = 2.7
  dimension "d1253" = 0.25
  constraint horizontal L0
  constraint vertical L1
  constraint horizontal L2
  constraint vertical L3
  measures "d1250" horizontal distance of origin L0.start
  measures "d1251" vertical distance of origin L0.start
  measures "d1252" horizontal distance of L0.start L0.end
  measures "d1253" vertical distance of L0.end L1.end
extrude "USB contact visual stripe (13)" add sketch "USB contact visual stripe sketch (13)" along normal blind 0.03 separate body makes body 56 in component "USB — contact detail — illustrative only"
ref_plane "WorkPlane15" through (0, 0, 27.35) normal (0, 0, 1) x (1, 0, 0) in component "USB — contact detail — illustrative only"
sketch "USB contact visual stripe sketch (14)" plane through (0, 0, 27.35) normal (0, 0, 1) x (1, 0, 0) in component "USB — contact detail — illustrative only"
  line L0 (71, 17.125) -> (73.7, 17.125)
  line L1 (73.7, 17.125) -> (73.7, 17.375)
  line L2 (73.7, 17.375) -> (71, 17.375)
  line L3 (71, 17.375) -> (71, 17.125)
  dimension "d1258" = 71
  dimension "d1259" = 17.125
  dimension "d1260" = 2.7
  dimension "d1261" = 0.25
  constraint horizontal L0
  constraint vertical L1
  constraint horizontal L2
  constraint vertical L3
  measures "d1258" horizontal distance of origin L0.start
  measures "d1259" vertical distance of origin L0.start
  measures "d1260" horizontal distance of L0.start L0.end
  measures "d1261" vertical distance of L0.end L1.end
extrude "USB contact visual stripe (14)" add sketch "USB contact visual stripe sketch (14)" along normal blind 0.03 separate body makes body 57 in component "USB — contact detail — illustrative only"
ref_plane "WorkPlane16" through (0, 0, 27.35) normal (0, 0, 1) x (1, 0, 0) in component "USB — contact detail — illustrative only"
sketch "USB contact visual stripe sketch (15)" plane through (0, 0, 27.35) normal (0, 0, 1) x (1, 0, 0) in component "USB — contact detail — illustrative only"
  line L0 (71, 17.625) -> (73.7, 17.625)
  line L1 (73.7, 17.625) -> (73.7, 17.875)
  line L2 (73.7, 17.875) -> (71, 17.875)
  line L3 (71, 17.875) -> (71, 17.625)
  dimension "d1266" = 71
  dimension "d1267" = 17.625
  dimension "d1268" = 2.7
  dimension "d1269" = 0.25
  constraint horizontal L0
  constraint vertical L1
  constraint horizontal L2
  constraint vertical L3
  measures "d1266" horizontal distance of origin L0.start
  measures "d1267" vertical distance of origin L0.start
  measures "d1268" horizontal distance of L0.start L0.end
  measures "d1269" vertical distance of L0.end L1.end
extrude "USB contact visual stripe (15)" add sketch "USB contact visual stripe sketch (15)" along normal blind 0.03 separate body makes body 58 in component "USB — contact detail — illustrative only"
ref_plane "WorkPlane1" through (0, 0, -4) normal (0, 0, 1) x (1, 0, 0) in component "M2 x 4 socket_cap screw — GEN-M2-SHCS-L4-AF1.5"
sketch "Joined screw sketch (4)" plane through (0, 0, -4) normal (0, 0, 1) x (1, 0, 0) in component "M2 x 4 socket_cap screw — GEN-M2-SHCS-L4-AF1.5"
  circle A0 centre (0, 0) radius 0.95
  dimension "d1274" = 0.95
  measures "d1274" radius of A0
extrude "Joined screw'''" add sketch "Joined screw sketch (4)" along normal blind 4 separate body makes body 59 in component "M2 x 4 socket_cap screw — GEN-M2-SHCS-L4-AF1.5"
ref_plane "WorkPlane2" through (0, 0, 0) normal (0, 0, 1) x (1, 0, 0) in component "M2 x 4 socket_cap screw — GEN-M2-SHCS-L4-AF1.5"
sketch "Screw head sketch (4)" plane through (0, 0, 0) normal (0, 0, 1) x (1, 0, 0) in component "M2 x 4 socket_cap screw — GEN-M2-SHCS-L4-AF1.5"
  circle A0 centre (0, 0) radius 1.9
  dimension "d1279" = 1.9
  measures "d1279" radius of A0
extrude "Screw head'''" add sketch "Screw head sketch (4)" along normal blind 2 bodies 59 in component "M2 x 4 socket_cap screw — GEN-M2-SHCS-L4-AF1.5"
fillet "Rounded head crown'''" radius 0.15 1 edges at (-1.7714, -0.6871, 2) on bodies 59 in component "M2 x 4 socket_cap screw — GEN-M2-SHCS-L4-AF1.5"
ref_plane "WorkPlane3" through (0, 0, 1) normal (0, 0, 1) x (1, 0, 0) in component "M2 x 4 socket_cap screw — GEN-M2-SHCS-L4-AF1.5"
sketch "Hex drive 1.5 mm across flats (3)" plane through (0, 0, 1) normal (0, 0, 1) x (1, 0, 0) in component "M2 x 4 socket_cap screw — GEN-M2-SHCS-L4-AF1.5"
  line L0 (0.866, 0) -> (0.433, 0.75)
  line L1 (0.433, 0.75) -> (-0.433, 0.75)
  line L2 (-0.433, 0.75) -> (-0.866, 0)
  line L3 (-0.866, 0) -> (-0.433, -0.75)
  line L4 (-0.433, -0.75) -> (0.433, -0.75)
  line L5 (0.433, -0.75) -> (0.866, 0)
extrude "Hex drive recess'''" cut sketch "Hex drive 1.5 mm across flats (3)" along normal blind 1.1 bodies 59 in component "M2 x 4 socket_cap screw — GEN-M2-SHCS-L4-AF1.5"
ref_plane "WorkPlane1" through (0, 0, -6) normal (0, 0, 1) x (1, 0, 0) in component "M2 x 6 socket_cap screw — GEN-M2-SHCS-L6-AF1.5"
sketch "Joined screw sketch (5)" plane through (0, 0, -6) normal (0, 0, 1) x (1, 0, 0) in component "M2 x 6 socket_cap screw — GEN-M2-SHCS-L6-AF1.5"
  circle A0 centre (0, 0) radius 0.95
  dimension "d1290" = 0.95
  measures "d1290" radius of A0
extrude "Joined screw''''" add sketch "Joined screw sketch (5)" along normal blind 6 separate body makes body 60 in component "M2 x 6 socket_cap screw — GEN-M2-SHCS-L6-AF1.5"
ref_plane "WorkPlane2" through (0, 0, 0) normal (0, 0, 1) x (1, 0, 0) in component "M2 x 6 socket_cap screw — GEN-M2-SHCS-L6-AF1.5"
sketch "Screw head sketch (5)" plane through (0, 0, 0) normal (0, 0, 1) x (1, 0, 0) in component "M2 x 6 socket_cap screw — GEN-M2-SHCS-L6-AF1.5"
  circle A0 centre (0, 0) radius 1.9
  dimension "d1295" = 1.9
  measures "d1295" radius of A0
extrude "Screw head''''" add sketch "Screw head sketch (5)" along normal blind 2 bodies 60 in component "M2 x 6 socket_cap screw — GEN-M2-SHCS-L6-AF1.5"
fillet "Rounded head crown''''" radius 0.15 1 edges at (-1.7714, -0.6871, 2) on bodies 60 in component "M2 x 6 socket_cap screw — GEN-M2-SHCS-L6-AF1.5"
ref_plane "WorkPlane3" through (0, 0, 1) normal (0, 0, 1) x (1, 0, 0) in component "M2 x 6 socket_cap screw — GEN-M2-SHCS-L6-AF1.5"
sketch "Hex drive 1.5 mm across flats (4)" plane through (0, 0, 1) normal (0, 0, 1) x (1, 0, 0) in component "M2 x 6 socket_cap screw — GEN-M2-SHCS-L6-AF1.5"
  line L0 (0.866, 0) -> (0.433, 0.75)
  line L1 (0.433, 0.75) -> (-0.433, 0.75)
  line L2 (-0.433, 0.75) -> (-0.866, 0)
  line L3 (-0.866, 0) -> (-0.433, -0.75)
  line L4 (-0.433, -0.75) -> (0.433, -0.75)
  line L5 (0.433, -0.75) -> (0.866, 0)
extrude "Hex drive recess''''" cut sketch "Hex drive 1.5 mm across flats (4)" along normal blind 1.1 bodies 60 in component "M2 x 6 socket_cap screw — GEN-M2-SHCS-L6-AF1.5"
ref_plane "WorkPlane32" through (0, 0, 37.2) normal (0, 0, 1) x (1, 0, 0) in component "01 Tapered printed housing"